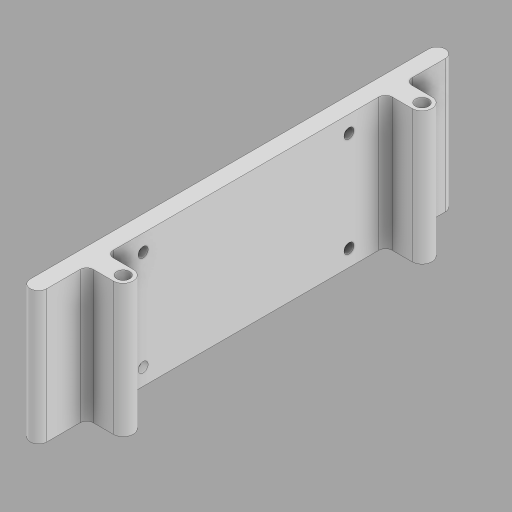
# Autodesk Inventor part: pod_akkum_2
Saved by Autodesk Inventor 2024.2 (Build 282272000, 272)
## iProperties
Created: 2024-02-18
Part Number: pod_akkum_2
Material: Типовые
Document SubType Name: Modeling
Designer: Fedor Orlov
Density: 1 g/cm^3
Appearance: По умолчанию
Author: Fedor Orlov
Autodesk Inventor part; units mm, degrees
ref_plane "YZ Plane" through (0, 0, 0) normal (1, 0, 0) x (0, 1, 0)
ref_plane "XZ Plane" through (0, 0, 0) normal (0, 1, 0) x (-1, 0, 0)
sketch "Эскиз1" plane through (0, 0, 0) normal (0, 1, 0) x (-1, 0, 0)
  line L0 (0, 45) -> (0, -45) construction
  circle A0 centre (0, 45) radius 1.5
  circle A1 centre (0, -45) radius 1.5
  line L1 (10.5, 60) -> (10.5, -60) construction
  line L2 (10.5, -60) -> (10.5, 60) construction
  line L3 (13, -60) -> (13, 60)
  line L4 (8, 60) -> (8, 48)
  arc A2 (8, -60) -> (13, -60) centre (10.5, -60) ccw
  arc A3 (13, 60) -> (8, 60) centre (10.5, 60) ccw
  arc A4 (0, 42) -> (0, 48) centre (0, 45) ccw construction
  arc A5 (0, -48) -> (0, -42) centre (0, -45) ccw construction
  line L5 (0, 48) -> (8, 48)
  line L6 (0, 42) -> (8, 42)
  line L7 (0, -42) -> (8, -42)
  line L8 (0, -48) -> (8, -48)
  arc A6 (0, -42) -> (0, -48) centre (0, -45) ccw
  arc A7 (0, 48) -> (0, 42) centre (0, 45) ccw
  line L9 (8, -42) -> (8, -48) construction
  line L10 (8, 42) -> (8, -42)
  line L11 (8, -48) -> (8, -60)
  line L12 (8, 48) -> (8, 42) construction
  point P0 (0, 0)
  point P1 (0, 0)
  point P2 (10.5, 0)
  dimension "d0" = 90
  dimension "d1" = 3
  dimension "d2" = 3
  dimension "d3" = 120
  dimension "d4" = 10.5
  dimension "d5" = 0
  dimension "d6" = 5
  dimension "d7" = 6
  dimension "d8" = 6
  constraints: 28 end point, 16 tangent, 15 perpendicular, 12 point on circle, 8 centre point, 6 parallel, 5 coincident, 3 midpoint, 3 point on line, 2 vertical, 1 collinear
  measures "d0" distance of L0.start L0.end
  measures "d1" diameter of A0
  measures "d2" diameter of A1
  measures "d3" distance of L1.start L1.end
  measures "d4" distance between parallel lines of L1 L0
  measures "d5" vertical distance of point (0, 0) point (10.5, 0)
  measures "d6" diameter of A3
  measures "d7" diameter of A4
  measures "d8" diameter of A5
extrude "Выдавливание1" add sketch "Эскиз1" along normal blind 40
fillet "Сопряжение1" radius 2 4 edges at (-8, 20, 42) (-8, 20, 48) (-8, 20, -42) (-8, 20, -48)
sketch "Эскиз2" plane through (0, 40, 0) normal (0, 1, 0) x (1, 0, 0)
  line L0 (0, 48) -> (-6, 48) projected
  arc A0 (-8, 50) -> (-6, 48) centre (-6, 50) ccw projected
  line L1 (-8, 50) -> (-8, 60) projected
  arc A1 (-8, 60) -> (-13, 60) centre (-10.5, 60) ccw projected
  line L2 (-13, 60) -> (-13, -60) projected
  arc A2 (-13, -60) -> (-8, -60) centre (-10.5, -60) ccw projected
  line L3 (-8, -60) -> (-8, -50) projected
  arc A3 (-6, -48) -> (-8, -50) centre (-6, -50) ccw projected
  line L4 (-6, -48) -> (0, -48) projected
  arc A4 (0, -48) -> (0, -42) centre (0, -45) ccw projected
  line L5 (0, -42) -> (-6, -42) projected
  arc A5 (-8, -40) -> (-6, -42) centre (-6, -40) ccw projected
  line L6 (-8, -40) -> (-8, 40) projected
  arc A6 (-6, 42) -> (-8, 40) centre (-6, 40) ccw projected
  line L7 (-6, 42) -> (0, 42) projected
  arc A7 (0, 42) -> (0, 48) centre (0, 45) ccw projected
  circle A8 centre (0, -45) radius 1.5 projected
  circle A9 centre (0, 45) radius 1.5 projected
  circle A10 centre (0, -45) radius 1.95
  circle A11 centre (0, 45) radius 1.95
  point P0 (0, 0)
  dimension "d12" = 3.9
  dimension "d13" = 3.9
  constraints: 2 centre point, 2 coincident
  measures "d12" diameter of A10
  measures "d13" diameter of A11
extrude "Выдавливание2" cut sketch "Эскиз2" against normal blind 4 contours A8 | A9 | A10 | A11
ref_plane "РабПлоскость1" through (0, 20, 0) normal (0, 1, 0) x (1, 0, 0)
mirror "Зеркальное отражение1" about plane through (0, 20, 0) normal (0, 1, 0) of "Выдавливание2"
sketch "Эскиз3" plane through (-8, 0, 40) normal (1, 0, 0) x (0, 0, -1)
  line L0 (40, 0) -> (40, 40) construction
  line L1 (0, 40) -> (80, 40) projected
  line L2 (71, 5) -> (9, 5) construction
  line L3 (9, 5) -> (9, 35) construction
  line L4 (9, 35) -> (71, 35) construction
  line L5 (71, 35) -> (71, 5) construction
  line L6 (71, 5) -> (9, 35) construction
  line L7 (9, 5) -> (71, 35) construction
  circle A0 centre (9, 35) radius 1.5
  circle A1 centre (71, 35) radius 1.5
  circle A2 centre (9, 5) radius 1.5
  circle A3 centre (71, 5) radius 1.5
  point P0 (40, 20)
  dimension "d17" = 62
  dimension "d18" = 30
  dimension "d19" = 3
  dimension "d20" = 3
  dimension "d21" = 3
  dimension "d22" = 3
  constraints: 14 end point, 4 centre point, 4 coincident, 4 midpoint, 2 parallel, 1 horizontal, 1 perpendicular
  measures "d17" distance of L3.end L4.end
  measures "d18" distance of L2.end L3.end
  measures "d19" diameter of A0
  measures "d20" diameter of A1
  measures "d21" diameter of A2
  measures "d22" diameter of A3
extrude "Выдавливание3" cut sketch "Эскиз3" against normal through all
sketch "Эскиз4" plane through (-13, 0, -60) normal (-1, 0, 0) x (0, 0, 1)
  circle A0 centre (29, 35) radius 1.5 projected
  circle A1 centre (91, 35) radius 1.5 projected
  line L0 (29, 35) -> (91, 35) construction
  circle A2 centre (91, 5) radius 1.5 projected
  line L1 (91, 35) -> (91, 5) construction
  line L2 (91, 20) -> (60, 20) construction
  line L3 (60, 20) -> (60, 35) construction
  line L4 (31.9, 36.6743) -> (31.9, 33.3257)
  line L5 (31.9, 33.3257) -> (29, 31.6514)
  line L6 (29, 31.6514) -> (26.1, 33.3257)
  line L7 (26.1, 33.3257) -> (26.1, 36.6743)
  line L8 (26.1, 36.6743) -> (29, 38.3486)
  line L9 (29, 38.3486) -> (31.9, 36.6743)
  circle A3 centre (29, 5) radius 1.5
  line L10 (31.9, 3.3257) -> (31.9, 6.6743)
  line L11 (31.9, 6.6743) -> (29, 8.3486)
  line L12 (29, 8.3486) -> (26.1, 6.6743)
  line L13 (26.1, 6.6743) -> (26.1, 3.3257)
  line L14 (26.1, 3.3257) -> (29, 1.6514)
  line L15 (29, 1.6514) -> (31.9, 3.3257)
  line L16 (91, 38.3486) -> (93.9, 36.6743)
  line L17 (93.9, 36.6743) -> (93.9, 33.3257)
  line L18 (93.9, 33.3257) -> (91, 31.6514)
  line L19 (91, 31.6514) -> (88.1, 33.3257)
  line L20 (88.1, 33.3257) -> (88.1, 36.6743)
  line L21 (88.1, 36.6743) -> (91, 38.3486)
  circle A4 centre (91, 5) radius 1.5
  line L22 (91, 1.6514) -> (93.9, 3.3257)
  line L23 (93.9, 3.3257) -> (93.9, 6.6743)
  line L24 (93.9, 6.6743) -> (91, 8.3486)
  line L25 (91, 8.3486) -> (88.1, 6.6743)
  line L26 (88.1, 6.6743) -> (88.1, 3.3257)
  line L27 (88.1, 3.3257) -> (91, 1.6514)
  point P0 (60, 0)
  dimension "d25" = 31
  dimension "d26" = 5.8
  dimension "d27" = 5.8
  dimension "d28" = 5.8
  dimension "d29" = 5.8
  constraints: 56 end point, 15 symmetric about line, 4 coincident, 2 centre point, 2 horizontal, 2 midpoint, 1 perpendicular, 28 other
  measures "d25" distance of L2.start L2.end
  measures "d26" distance between parallel lines of L6 L9
  measures "d27" horizontal distance of L4.start L6.end
  measures "d28" distance between parallel lines of L17 L20
  measures "d29" horizontal distance of L16.end L19.end
extrude "Выдавливание4" cut sketch "Эскиз4" against normal blind 3 contours A0 | A1 | A2 | L4 L5 L6 L7 L8 L9 | A3 | L15 L14 L13 L12 L11 L10 | L16 L17 L18 L19 L20 L21 | L27 L26 L25 L24 L23 L22
equation "\"d8\" = d7"
